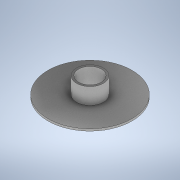
# Autodesk Inventor part: motor platform reaction wheel
Saved by Autodesk Inventor 2021 (Build 250183000, 183)
## iProperties
Created: 2021-07-29
Part Number: motor platform reaction wheel
Material: ABS Plastic
Document SubType Name: Modeling
Designer: samlo
Density: 1.06 g/cm^3
Appearance: Honed
Author: samlo
Autodesk Inventor part; units mm, degrees
ref_plane "YZ Plane" through (0, 0, 0) normal (1, 0, 0) x (0, 1, 0)
ref_plane "XZ Plane" through (0, 0, 0) normal (0, 1, 0) x (-1, 0, 0)
ref_plane "XY Plane" through (0, 0, 0) normal (0, 0, 1) x (1, 0, 0)
sketch "Sketch1" plane through (0, 0, 0) normal (0, 0, 1) x (1, 0, 0)
  line L0 (4, 0) -> (7, 0)
  line L1 (7, 0) -> (7, 8)
  line L2 (7, 8) -> (51.45, 8)
  line L3 (51.45, 8) -> (51.45, 10.5)
  line L4 (4, 8) -> (4, 0)
  line L5 (0, 10.5) -> (0, 8)
  line L6 (0, 8) -> (4, 8)
  line L7 (0, 10.5) -> (13.95, 10.5)
  line L8 (13.95, 10.5) -> (13.95, 30.5)
  line L9 (13.95, 30.5) -> (16.45, 30.5)
  line L10 (16.45, 30.5) -> (16.45, 10.5)
  line L11 (16.45, 10.5) -> (51.45, 10.5)
  point P0 (0, 0)
  dimension "d0" = 4
  dimension "d1" = 8
  dimension "d2" = 0
  dimension "d3" = 2.5
  dimension "d4" = 3
  dimension "d7" = 2.5
  dimension "d8" = 35
  dimension "d9" = 13.95
  dimension "d10" = 20
  constraints: 24 end point, 8 perpendicular, 2 horizontal, 2 point on line
  measures "d0" distance of L5.end L4.start
  measures "d1" distance of L4.start L0.start
  measures "d2" distance from line of point (0, 0) L0
  measures "d3" distance of L5.start L5.end
  measures "d4" distance of L0.start L0.end
  measures "d7" distance of L8.end L9.end
  measures "d8" distance of L10.end L3.end
  measures "d9" distance of L5.start L7.end
  measures "d10" distance of L7.end L8.end
revolve "Revolution1" add sketch "Sketch1" angle 360 about axis through (0, 10.5, 0) along (0, -1, 0)
thread "Thread1" size "M8x1.25" class "6H" standard "ANSI Metric M Profile" full length
body "Solid1"
